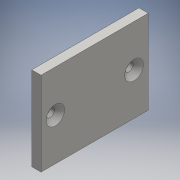
# Autodesk Inventor part: coperchietto
Saved by Autodesk Inventor 2016 (Build 200138000, 138)
## iProperties
Created: 2017-11-07
Part Number: coperchietto
Material: Generic
Document SubType Name: Modeling
Designer: Davide
Density: 1 g/cm^3
Appearance: Default
Author: Davide
Autodesk Inventor part; units mm, degrees
ref_plane "YZ Plane" through (0, 0, 0) normal (1, 0, 0) x (0, 1, 0)
ref_plane "XZ Plane" through (0, 0, 0) normal (0, 1, 0) x (-1, 0, 0)
ref_plane "XY Plane" through (0, 0, 0) normal (0, 0, 1) x (1, 0, 0)
sketch "Sketch1" plane through (0, 0, 0) normal (1, 0, 0) x (0, 1, 0)
  line L0 (-12.4, 9) -> (10.6, 9)
  line L1 (10.6, 9) -> (10.6, -9)
  line L2 (10.6, -9) -> (-12.4, -9)
  line L3 (-12.4, -9) -> (-12.4, 9)
  circle A0 centre (7.55, 0) radius 0.9
  circle A1 centre (-9.35, 0) radius 0.9
  line L4 (-0.9, 9) -> (-0.9, -9) construction
  line L5 (8.45, 0) -> (-10.25, 0) construction
  point P0 (-0.9, 0)
  point P1 (-0.9, 0)
  dimension "d5" = 1.8
  dimension "d6" = 1.8
  dimension "d0" = 23
  dimension "d1" = 18
  dimension "d4" = 16.9
  constraints: 12 end point, 7 midpoint, 3 perpendicular, 3 point on line, 2 horizontal alignment, 2 parallel, 1 horizontal, 4 other
  measures "d0" distance of L1.end L2.end
  measures "d1" distance of L1.end L0.end
  measures "d4" distance of point (-9.35, 0) point (7.55, 0)
extrude "Extrusion1" add sketch "Sketch1" along normal blind 2
hole "Hole1" at (2, 7.55, 0) direction (-1, 0, 0) diameter 1.8 depth 15 tip angle 118 countersink diameter 4 countersink angle 90
hole "Hole2" at (2, -9.3379, 0.0682) direction (-1, 0, 0) diameter 1.8 depth 15 tip angle 118 countersink diameter 4 countersink angle 90
equation "\"d6\" = d5"
body "Solid1"
